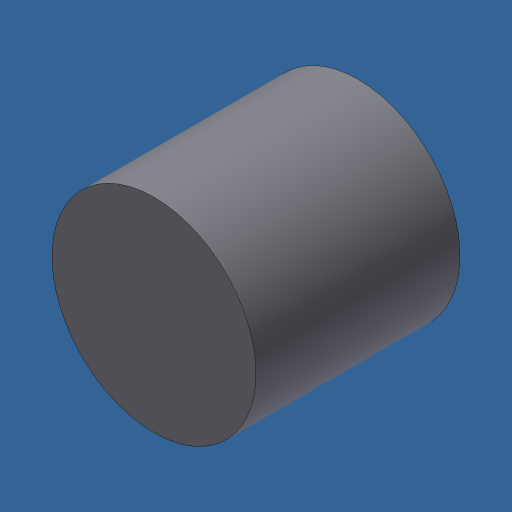
# Autodesk Inventor part: Cylinder, Center Constrained (mm)
Saved by Autodesk Inventor 2024.3 (Build 283343000, 343)
## iProperties
Category: _
Manager: _
Created: 2023-11-08
Part Number: Cylinder, Center Constrained (mm)
Checked By: 00
Engr Approved By: _
User Status: Work In Process
Material: Steel, MS
Description: CYLINDER, CENTER CONSTRAINED (mm).ipt
Document SubType Name: Modeling
Mfg Approved By: Stephen.Oerton
Designer: Raamprakash.Soundaran
Manufacturer: Standard
Standards Organization: Custom
Mass: 192.913 g
Surface Area: 49.0874 cm^2
Volume: 24.5437 cm^3
Density: 7.86 g/cm^3
Appearance: Metal-Steel
CN_MASS: 0.19
PTC_WM_ITERATION: 2
PTC_WM_ORGANIZATION_ID: CLWC
PTC_WM_LIFECYCLE: CLWC_CAD_LC
CN_SERVICEABLE: _
CL_runCount: 0
FIRST_DESCRIPTION: _
SECOND_DESCRIPTION: _
THIRD_DESCRIPTION: _
ModelCat: Uncategorized
ILogicPurgeVersion: 2.2.20.20
OnSaveVersion: 2.2.20.30
Subject: _
Author: Raamprakash.Soundaran
Keywords: -
Revision Number: B
Autodesk Inventor part; units mm, degrees
ref_plane "YZ Plane" through (0, 0, 0) normal (1, 0, 0) x (0, 1, 0)
ref_plane "XZ Plane" through (0, 0, 0) normal (0, 1, 0) x (-1, 0, 0)
ref_plane "XY Plane" through (0, 0, 0) normal (0, 0, 1) x (1, 0, 0)
sketch "Sketch2" plane through (0, 0, 0) normal (1, 0, 0) x (0, 1, 0)
  line L0 (0, 12.5) -> (-12.5, 12.5)
  line L1 (-12.5, 12.5) -> (-12.5, -12.5)
  line L2 (-12.5, -12.5) -> (0, -12.5)
  line L3 (0, -12.5) -> (0, 12.5)
  point P0 (0, 0)
  point P1 (0, 0)
  dimension "d4" = 25
  dimension "d7" = 25
  constraints: 9 end point, 2 midpoint, 2 parallel, 1 coincident, 1 perpendicular, 1 vertical
  measures "d4" distance of L0.end L1.end
  measures "d7" diameter of L1 L3
revolve "Revolution1" add sketch "Sketch2" angle 360 about axis through (0, 0, -12.5) along (0, 0, 1)
